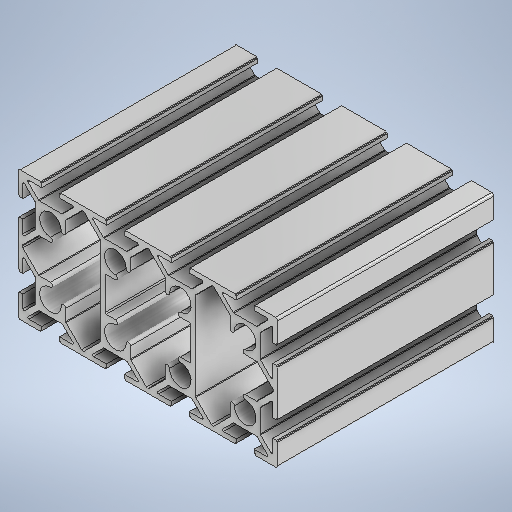
# Autodesk Inventor part: Perfil 60×120 12 rasgos_001
Saved by Autodesk Inventor 2026 (Build 300175000, 175)
## iProperties
Created: 2025-04-06
Part Number: Perfil 60×120 12 rasgos_001
Material: Aluminum 6061
Document SubType Name: Modeling
Designer: Tony Dias
Density: 2.7 g/cm^3
Appearance: Aluminum - Polished
Author: Tony Dias
Autodesk Inventor part; units mm, degrees
ref_plane "YZ Plane" through (0, 0, 0) normal (1, 0, 0) x (0, 1, 0)
ref_plane "XZ Plane" through (0, 0, 0) normal (0, 1, 0) x (-1, 0, 0)
ref_plane "XY Plane" through (0, 0, 0) normal (0, 0, 1) x (1, 0, 0)
sketch "Sketch1" plane through (0, 0, 0) normal (0, 0, 1) x (1, 0, 0)
  circle A0 centre (-45, 15) radius 5 construction
  circle A1 centre (-15, 15) radius 5 construction
  line L0 (-60, 30) -> (-60, 19.1) construction
  line L1 (-60, 30) -> (-49.1, 30) construction
  line L2 (-60, 19.1) -> (-57.8, 19.1) construction
  line L3 (-60, 30) -> (-45, 15) construction
  line L4 (-52, 22) -> (-52, 8) construction
  line L5 (-45, 15) -> (-45, 30) construction
  line L6 (-45, 15) -> (-30, 30) construction
  line L7 (-40.9, 30) -> (-30, 30) construction
  line L8 (-15, 15) -> (-30, 30) construction
  line L9 (-15, 15) -> (0, 30) construction
  line L10 (-30, 30) -> (-19.1, 30) construction
  line L11 (-49.1, 30) -> (-49.1, 27.8) construction
  line L12 (-40.9, 30) -> (-40.9, 27.8) construction
  line L13 (-52, 22) -> (-38, 22) construction
  line L14 (-56.2444, 27.8) -> (-50.4444, 22)
  line L15 (-56.2444, 27.8) -> (-49.1, 27.8)
  line L16 (-57.8, 26.2444) -> (-52, 20.4444)
  line L17 (-57.8, 26.2444) -> (-57.8, 19.1)
  line L18 (-52, 8) -> (-38, 8) construction
  line L19 (-38, 8) -> (-38, 22) construction
  line L20 (-60, 0) -> (-45, 15) construction
  line L21 (-57.8, 3.7556) -> (-52, 9.5556)
  line L22 (-57.8, 3.7556) -> (-57.8, 10.9)
  line L23 (-57.8, 10.9) -> (-60, 10.9) construction
  line L24 (-60, 10.9) -> (-60, 0) construction
  line L25 (-50.4444, 8) -> (-57.8, 0.6444)
  arc A2 (-57.8, 0.6444) -> (-58.0909, 0) centre (-57.0929, -0.0627) ccw
  line L26 (-60, 0) -> (-58.0909, 0)
  line L27 (-52, 20.4444) -> (-52, 9.5556)
  line L28 (-50.4444, 8) -> (-45, 8)
  line L29 (-33.7556, 27.8) -> (-39.5556, 22)
  line L30 (-33.7556, 27.8) -> (-40.9, 27.8)
  line L31 (-39.5556, 22) -> (-50.4444, 22)
  line L32 (-30.6444, 27.8) -> (-38, 20.4444)
  line L33 (-38, 20.4444) -> (-38, 15)
  arc A3 (-40, 15) -> (-45, 10) centre (-45, 15) ccw
  arc A4 (-45, 8) -> (-45, 10) centre (-45, 9) ccw
  arc A5 (-40, 15) -> (-38, 15) centre (-39, 15) ccw
  line L34 (-22, 22) -> (-8, 22) construction
  line L35 (-22, 22) -> (-22, 0) construction
  line L36 (-8, 22) -> (-8, 15) construction
  line L37 (-19.8, 8) -> (-19.8, 0)
  line L38 (-19.8, 0) -> (-22, 0)
  line L39 (-19.8, 8) -> (-15, 8)
  arc A6 (-10, 15) -> (-15, 10) centre (-15, 15) ccw
  arc A7 (-15, 8) -> (-15, 10) centre (-15, 9) ccw
  arc A8 (-10, 15) -> (-8, 15) centre (-9, 15) ccw
  line L40 (-29.3556, 27.8) -> (-22, 20.4444)
  arc A9 (-29.3556, 27.8) -> (-30.6444, 27.8) centre (-30, 27.0353) ccw
  line L41 (-26.2444, 27.8) -> (-20.4444, 22)
  line L42 (-26.2444, 27.8) -> (-19.1, 27.8)
  line L43 (-19.1, 27.8) -> (-19.1, 30) construction
  line L44 (-22, 20.4444) -> (-22, 0)
  line L45 (-3.7556, 27.8) -> (-9.5556, 22)
  line L46 (-3.7556, 27.8) -> (-10.9, 27.8)
  line L47 (-10.9, 27.8) -> (-10.9, 30) construction
  line L48 (-8, 20.4444) -> (-0.6444, 27.8)
  arc A10 (0, 28.0909) -> (-0.6444, 27.8) centre (0.0627, 27.0929) ccw
  line L49 (-10.9, 30) -> (0, 30) construction
  line L50 (0, 30) -> (0, 28.0909)
  line L51 (-8, 15) -> (-8, 20.4444)
  line L52 (-9.5556, 22) -> (-20.4444, 22)
  line L53 (-60, 10.9) -> (-59.5, 10.9) construction
  line L54 (-59.5, 10.9) -> (-59.5, 10.4)
  line L55 (-59.5, 10.4) -> (-60, 10.4)
  line L56 (-60, 10.4) -> (-60, 10.9) construction
  line L57 (-59.5, 10.9) -> (-57.8, 10.9)
  line L58 (-60, 10.4) -> (-60, 0)
  line L59 (-60, 19.1) -> (-59.5, 19.1) construction
  line L60 (-59.5, 19.1) -> (-59.5, 19.6)
  line L61 (-59.5, 19.6) -> (-60, 19.6)
  line L62 (-60, 19.6) -> (-60, 19.1) construction
  line L63 (-59.5, 19.1) -> (-57.8, 19.1)
  line L64 (-60, 30) -> (-60, 19.6)
  line L65 (-49.1, 30) -> (-49.6, 30) construction
  line L66 (-49.6, 30) -> (-49.6, 29.5)
  line L67 (-49.6, 29.5) -> (-49.1, 29.5)
  line L68 (-49.1, 29.5) -> (-49.1, 30) construction
  line L69 (-49.1, 29.5) -> (-49.1, 27.8)
  line L70 (-49.6, 30) -> (-60, 30)
  line L71 (-40.9, 30) -> (-40.4, 30) construction
  line L72 (-40.4, 30) -> (-40.4, 29.5)
  line L73 (-40.4, 29.5) -> (-40.9, 29.5)
  line L74 (-40.9, 29.5) -> (-40.9, 30) construction
  line L75 (-40.9, 29.5) -> (-40.9, 27.8)
  line L76 (-19.1, 30) -> (-19.6, 30) construction
  line L77 (-19.6, 30) -> (-19.6, 29.5)
  line L78 (-19.6, 29.5) -> (-19.1, 29.5)
  line L79 (-19.1, 29.5) -> (-19.1, 30) construction
  line L80 (-19.1, 29.5) -> (-19.1, 27.8)
  line L81 (-19.6, 30) -> (-40.4, 30)
  line L82 (-10.9, 30) -> (-10.4, 30) construction
  line L83 (-10.4, 30) -> (-10.4, 29.5)
  line L84 (-10.4, 29.5) -> (-10.9, 29.5)
  line L85 (-10.9, 29.5) -> (-10.9, 30) construction
  line L86 (-10.9, 29.5) -> (-10.9, 27.8)
  line L87 (-10.4, 30) -> (0, 30)
  line L88 (0, 30) -> (0, 28.0909)
  point P0 (0, 0)
  dimension "d0" = 10
  dimension "d2" = 15
  dimension "d3" = 45
  dimension "d4" = 10
  dimension "d5" = 15
  dimension "d6" = 60
  dimension "d7" = 30
  dimension "d8" = 4.1
  dimension "d10" = 4.1
  dimension "d11" = 2.2
  dimension "d12" = 8
  dimension "d13" = 1.1
  dimension "d14" = 2.2
  dimension "d15" = 1.1
  dimension "d16" = 1
  dimension "d18" = 2.2
  dimension "d19" = 1.1
  dimension "d20" = 1.1
  dimension "d21" = 0.5
  constraints: 178 end point, 27 equal length, 22 point on circle, 19 horizontal, 18 collinear, 17 horizontal alignment, 16 point on line, 15 parallel, 13 vertical, 11 centre point, 8 tangent, 8 vertical alignment, 7 perpendicular, 4 equal radius, 4 midpoint, 7 other
  measures "d0" diameter of A0
  measures "d2" vertical distance of point (0, 0) L3.end
  measures "d3" horizontal distance of point (0, 0) L3.end
  measures "d4" diameter of A1
  measures "d5" horizontal distance of point (0, 0) L8.start
  measures "d6" horizontal distance of point (0, 0) L0.start
  measures "d7" vertical distance of point (0, 0) L0.start
  measures "d8" horizontal distance of L3.end L1.end
  measures "d10" vertical distance of L3.end L0.end
  measures "d11" distance of L0.end L2.end
  measures "d12" distance from line of L0.end L4
  measures "d13" distance between parallel lines of L3 L14
  measures "d14" distance from line of L1 L14.start
  measures "d15" distance between parallel lines of L20 L21
  measures "d16" radius of A2
  measures "d18" distance between parallel lines of L35 L37
  measures "d19" distance between parallel lines of L8 L40
  measures "d20" distance between parallel lines of L9 L45
  measures "d21" distance of L54.end L55.end
extrude "Extrusion1" add sketch "Sketch1" along normal mid plane 100
fillet "Fillet1" radius 1 1 edges at (-60, 30, 0)
fillet "Fillet2" radius 0.5 17 edges at (-50.4444, 22, 0) (-20.4444, 22, 0) (-39.5556, 22, 0) (-52, 9.5556, 0) (-52, 20.4444, 0) (-9.5556, 22, 0) (-22, 20.4444, 0) (-56.2444, 27.8, 0) (-26.2444, 27.8, 0) (-38, 20.4444, 0) (-19.8, 8, 0) (-8, 20.4444, 0) (-50.4444, 8, 0) (-3.7556, 27.8, 0) (-33.7556, 27.8, 0) (-57.8, 3.7556, 0) (-57.8, 26.2444, 0)
mirror "Mirror1" about plane through (0, 0, 0) normal (0, 1, 0) of "Extrusion1", "Fillet1", "Fillet2"
mirror "Mirror2" about plane through (0, 0, 0) normal (1, 0, 0) of "Extrusion1", "Fillet1", "Fillet2", "Mirror1"
equation "\"d10\" = d8"
equation "\"d14\" = d11"
equation "\"d15\" = d13"
equation "\"d18\" = d11"
equation "\"d19\" = d15"
equation "\"d20\" = d13"
body "Solid1"
